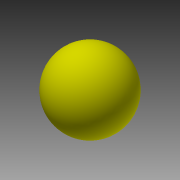
# Autodesk Inventor part: W 639/2-2Z_PART3
Saved by Autodesk Inventor 2014 SP2 (Build 180246200, 246)
## iProperties
Created: 2018-11-24
Part Number: W 639/2-2Z_PART3
Material: Generic
Catalog Web Link: www.cadenas.de
Description: -Deep groove ball bearings
Vendor: SKF
Document SubType Name: Modeling
Designer: psadmin
Manufacturer: SKF
Mass: 0.000904779 g
Surface Area: 0.0452389 cm^2
Volume: 0.000904779 cm^3
Density: 1 g/cm^3
Appearance: PSOLRGB-192-192-192
Category: PARTsolutions
Company: SKF
Title: W 639/2-2Z_PART3
Author: Cadenas PARTsolutions
Comments: Deep groove ball bearings
PSOL_IDENT_0: {$CADENAS_DATA\23d-libs\skf\bearings_units_and_housings\ball_bearings\deep_groove_ball_bearings\bb1_
PSOL_IDENT_1: 001_101.prj},199 {VTYP=3D},{NB=W 639/2-2Z_PART3},{LINA=W 639/2-2Z_PART3},{NN=BB1_001_101_PART3},{NOP
PSOL_IDENT_2: RJ=TRUE},{DATE=05.11.2018 07:58:23},{GEOMDATE=08.08.2018 12:16:40},{VERSION=},{LINEID=18460},{WBVAR=
PSOL_IDENT_3: },{WBNUMERIC=}  {NB=W 639/2-2Z_PART3},{LINA=W 639/2-2Z_PART3},{KT=DUMMY},{PRODUCTID=1010476392},{DES
PSOL_IDENT_4: IGNATION=W 639/2-2Z},{DD=2.00},{D=6.000},{B=3.000},{C=0.000},{DD1=3.00},{DD2=0.0},{D1=0.00},{D2=5.40
PSOL_IDENT_5: },{D3=0.00},{D4=0.000},{HH=MIN},{BB=0.000},{FF=0.00},{R0MAX=MIN},{R0=MIN},{R12=0.15},{PITCH=3.90},{D
PSOL_IDENT_6: W=1.200},{DDAMIN=2.900},{DDAMAX=2.900},{DDBMIN=MIN},{DDBMAX=MIN},{DBMIN=MIN},{DAMAX=5.400},{BBAMIN=M
PSOL_IDENT_7: IN},{CAMAX=MIN},{RAMAX=0.150},{LOAD1=0.190},{LOAD2=0.051},{LOAD3=0.002},{SPEED1=180000},{SPEED2=9000
PSOL_IDENT_8: 0},{KR=0.025},{F0=6.000},{Z=6},{II=1},{MASS=0.000},{BEARING=W 639/2-2Z},{RING=},{HELP=0.648},{HELP2=
PSOL_IDENT_9: 0.300},{DD1ALG=1.500},{YALG=1.500},{PITCH1=3.900},{DW1=1.200},{YALG1=2.352},{HALG1=0.648},{SH=1.500}
PSOL_IDENT_10: ,{CU=0.360},{DESIGN=dgbbw2z},{HALG=0.5},{B1=0},{ALGO=1.000}
NT: Deep groove ball bearings
NB: W 639/2-2Z_PART3
NBSYN: $DESIGNATION._PART3
LINA: W 639/2-2Z_PART3
SUPPLIER: SKF
ARTICLENO: W 639/2-2Z_PART3
BOMINFO: W 639/2-2Z_PART3
CREATOR: CADENAS GmbH
Autodesk Inventor part; units mm, degrees
ref_plane "YZ Plane" through (0, 0, 0) normal (1, 0, 0) x (0, 1, 0)
ref_plane "XZ Plane" through (0, 0, 0) normal (0, 1, 0) x (-1, 0, 0)
ref_plane "XY Plane" through (0, 0, 0) normal (0, 0, 1) x (1, 0, 0)
sketch "Sketch_6" plane through (0, 0, 0) normal (0, 0, 1) x (1, 0, 0)
  line L0 (2.1, 1.95) -> (0.9, 1.95)
  arc A0 (2.1, 1.95) -> (0.9, 1.95) centre (1.5, 1.95) ccw
  line L1 (2.1, 1.95) -> (0.9, 1.95)
  dimension "d0" = 360
  constraints: 4 end point, 2 point on circle, 1 centre point
revolve "Revolution1" add sketch "Sketch_6" angle 360 about axis through (2.1, 1.95, 0) along (1, 0, 0)
body "Solid1"
